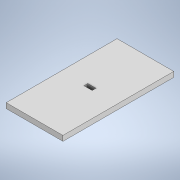
# Autodesk Inventor part: body
Saved by Autodesk Inventor 2022.1 (Build 261234020, 234B)
## iProperties
Created: 2021-10-31
Part Number: body
Material: Generic
Document SubType Name: Modeling
Designer: 46734
Density: 1 g/cm^3
Appearance: Default
Author: 46734
Autodesk Inventor part; units mm, degrees
ref_plane "YZ Plane" through (0, 0, 0) normal (1, 0, 0) x (0, 1, 0)
ref_plane "XZ Plane" through (0, 0, 0) normal (0, 1, 0) x (-1, 0, 0)
ref_plane "XY Plane" through (0, 0, 0) normal (0, 0, 1) x (1, 0, 0)
sketch "Sketch1" plane through (0, 0, 0) normal (0, 1, 0) x (-1, 0, 0)
  line L0 (0, 0) -> (110, 0)
  line L1 (110, 0) -> (110, -215)
  line L2 (110, -215) -> (0, -215)
  line L3 (0, -215) -> (0, 0)
  line L4 (62.9637, -103.7568) -> (47.0363, -103.7568)
  line L5 (47.0363, -103.7568) -> (47.0363, -111.2432)
  line L6 (47.0363, -111.2432) -> (62.9637, -111.2432)
  line L7 (62.9637, -111.2432) -> (62.9637, -103.7568)
  line L8 (62.9637, -103.7568) -> (47.0363, -111.2432) construction
  line L9 (47.0363, -103.7568) -> (62.9637, -111.2432) construction
  point P0 (55, -107.5)
  point P1 (55, -215)
  point P2 (55, -107.5)
  dimension "d0" = 110
  dimension "d1" = 215
  dimension "d4" = 103.7568
  dimension "d6" = 15.9273
  dimension "d7" = 47.0363
  dimension "d8" = 7.4865
  constraints: 20 end point, 4 midpoint, 4 parallel, 2 horizontal, 2 perpendicular
  measures "d0" distance of L1.end L2.end
  measures "d1" distance of L0.end L1.end
  measures "d4" distance between parallel lines of L2 L6
  measures "d6" distance of L4.start L4.end
  measures "d7" distance from line of L3 L4.end
  measures "d8" distance of L6.end L4.start
extrude "Extrusion1" add sketch "Sketch1" along normal blind 10
body "Solid1"
